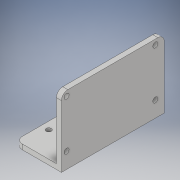
# Autodesk Inventor part: LimeLight90
Saved by Autodesk Inventor 2019 (Build 230136000, 136)
## iProperties
Created: 2019-12-14
Part Number: LimeLight90
Material: Generic
Document SubType Name: Modeling
Designer: james
Density: 1 g/cm^3
Appearance: Default
Author: james
Autodesk Inventor part; units mm, degrees
ref_plane "YZ Plane" through (0, 0, 0) normal (1, 0, 0) x (0, 1, 0)
ref_plane "XZ Plane" through (0, 0, 0) normal (0, 1, 0) x (-1, 0, 0)
ref_plane "XY Plane" through (0, 0, 0) normal (0, 0, 1) x (1, 0, 0)
sketch "Sketch1" plane through (0, 0, 0) normal (1, 0, 0) x (0, 1, 0)
  line L0 (44.4049, 39.363) -> (-19.0951, 39.363)
  line L1 (-19.0951, 39.363) -> (-19.0951, -63.507)
  line L2 (-19.0951, -63.507) -> (44.4049, -63.507)
  line L3 (44.4049, -63.507) -> (44.4049, 39.363)
  point P0 (0, 0)
  dimension "d0" = 102.87
  dimension "d1" = 63.5
  constraints: 8 end point, 2 parallel, 1 horizontal, 1 perpendicular
  measures "d0" distance of L0.end L1.end
  measures "d1" distance of L0.start L0.end
extrude "Extrusion1" add sketch "Sketch1" along normal blind 5.08
sketch "Sketch2" plane through (5.08, 0, 0) normal (1, 0, 0) x (0, 0, -1)
  line L0 (63.507, 44.4049) -> (-39.363, 44.4049) projected
  line L1 (-39.363, 44.4049) -> (-39.363, -19.0951) projected
  point P0 (0, 0)
  point P1 (-34.283, 39.3249)
  point P2 (54.617, 39.3249)
  point P3 (54.617, -8.3001)
  point P4 (-34.283, -8.3001)
  dimension "d4" = 0
  dimension "d5" = 0
  dimension "d6" = 0
  dimension "d7" = 0
  dimension "d8" = 88.9
  dimension "d9" = 5.08
  dimension "d10" = 5.08
  dimension "d11" = 47.625
  measures "d4" horizontal distance of point (-34.283, -8.3) point (-34.283, 39.325)
  measures "d5" horizontal distance of point (54.617, -8.3) point (54.617, 39.325)
  measures "d6" vertical distance of point (-34.283, 39.325) point (54.617, 39.325)
  measures "d7" vertical distance of point (-34.283, -8.3) point (54.617, -8.3)
  measures "d8" distance of point (54.617, 39.325) point (-34.283, 39.325)
  measures "d9" distance from line of L0 point (-34.283, 39.325)
  measures "d10" distance from line of L1 point (-34.283, 39.325)
  measures "d11" distance of point (-34.283, -8.3) point (-34.283, 39.325)
hole "Hole1" at (5.08, 39.3249, 34.283) at (5.08, 39.3249, -54.617) at (5.08, -8.3001, -54.617) at (5.08, -8.3001, 34.283) direction (-1, 0, 0) diameter 5.1054 end through all clearance for "Flat Head Machine Screw (82)" size "#10" standard "Ansi Unified Screw Threads"
sketch "Sketch3" plane through (0, -19.0951, -63.507) normal (0, -1, 0) x (1, 0, 0)
  line L0 (-45.72, 0) -> (5.08, 0)
  line L1 (5.08, 0) -> (5.08, 102.87)
  line L2 (5.08, 102.87) -> (-45.72, 102.87)
  line L3 (-45.72, 102.87) -> (-45.72, 0)
  line L4 (5.08, 102.87) -> (5.08, 0) projected
  line L5 (0, 0) -> (5.08, 0) projected
  line L6 (0, 102.87) -> (5.08, 102.87) projected
  point P0 (0, 63.507)
  dimension "d19" = 0
  dimension "d20" = 0
  dimension "d21" = 0
  dimension "d22" = 50.8
  constraints: 8 end point, 2 parallel, 1 horizontal, 1 perpendicular
  measures "d19" distance between parallel lines of L4 L1
  measures "d20" distance between parallel lines of L5 L0
  measures "d21" distance between parallel lines of L6 L2
  measures "d22" distance between parallel lines of L1 L3
extrude "Extrusion2" add sketch "Sketch3" along normal blind 5.08
sketch "Sketch4" plane through (0, -19.0951, -63.507) normal (0, 1, 0) x (1, 0, 0)
  line L0 (0, -102.87) -> (-45.72, -102.87) projected
  line L1 (-45.72, 0) -> (0, 0) projected
  line L2 (5.08, 0) -> (5.08, -102.87) projected
  point P0 (0, -63.507)
  point P1 (-7.62, -77.47)
  point P2 (-33.02, -77.47)
  point P3 (-33.02, -26.67)
  point P4 (-7.62, -26.67)
  dimension "d25" = 0
  dimension "d26" = 0
  dimension "d27" = 0
  dimension "d28" = 0
  dimension "d29" = 25.4
  dimension "d30" = 50.8
  dimension "d31" = 25.4
  dimension "d32" = 26.67
  dimension "d33" = 12.7
  measures "d25" horizontal distance of point (-7.62, -26.67) point (-7.62, -77.47)
  measures "d26" horizontal distance of point (-33.02, -26.67) point (-33.02, -77.47)
  measures "d27" vertical distance of point (-7.62, -77.47) point (-33.02, -77.47)
  measures "d28" vertical distance of point (-7.62, -26.67) point (-33.02, -26.67)
  measures "d29" distance of point (-7.62, -77.47) point (-33.02, -77.47)
  measures "d30" distance of point (-33.02, -26.67) point (-33.02, -77.47)
  measures "d31" distance from line of L0 point (-33.02, -77.47)
  measures "d32" distance from line of L1 point (-33.02, -26.67)
  measures "d33" distance from line of L2 point (-7.62, -26.67)
hole "Hole2" at (-7.62, -19.0951, 13.963) at (-33.02, -19.0951, 13.963) at (-33.02, -19.0951, -36.837) at (-7.62, -19.0951, -36.837) direction (0, -1, 0) diameter 5.1054 end through all clearance for "Flat Head Machine Screw (82)" size "#10" standard "Ansi Unified Screw Threads"
sketch "Sketch5" plane through (0, -24.1751, -63.507) normal (0, -1, 0) x (1, 0, 0)
  line L0 (-91.5665, 115.4463) -> (-40.64, 115.4463)
  line L1 (-40.64, 115.4463) -> (-40.64, -11.0997)
  line L2 (-40.64, -11.0997) -> (-91.5665, -11.0997)
  line L3 (-91.5665, -11.0997) -> (-91.5665, 115.4463)
  line L4 (-45.72, 102.87) -> (-45.72, 0) projected
  point P0 (0, 63.507)
  dimension "d41" = 5.08
  constraints: 8 end point, 2 parallel, 1 horizontal, 1 perpendicular
  measures "d41" distance between parallel lines of L4 L1
extrude "Extrusion3" cut sketch "Sketch5" against normal blind 25.4
fillet "Fillet1" radius 6.35 4 edges at (-40.64, -21.6351, -63.507) (-40.64, -21.6351, 39.363) (2.54, 44.4049, 39.363) (2.54, 44.4049, -63.507)
body "Solid1"
